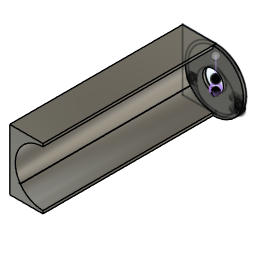
Sin+título(1) (Autodesk Fusion 360 design; units mm, degrees)
Autodesk Fusion 360 part; units mm, degrees
sketch "Boceto1" plane through (0, 0, 0) normal (0, 1, 0) x (1, 0, 0)
  circle A0 centre (0, 0) radius 14
  circle A1 centre (-17.5, 0) radius 2
  circle A2 centre (-17.5, 0) radius 3.5
  line L0 (-17.5, -3.5) -> (-13.5554, -3.5)
  line L1 (-17.5, 3.5) -> (-13.5554, 3.5)
  line L2 (0, -1.75) -> (0, -22.5)
  circle A3 centre (17.5, 0) radius 2
  circle A4 centre (17.5, 0) radius 3.5
  line L3 (17.5, 3.5) -> (13.5554, 3.5)
  line L4 (17.5, -3.5) -> (13.5554, -3.5)
  circle A5 centre (0, -8) radius 7.5
  circle A6 centre (0, -8) radius 20
  circle A7 centre (0, -8) radius 22
  line L5 (0, -30) -> (-24, -30)
  line L6 (-24, -30) -> (-24, 14)
  line L7 (-24, 14) -> (0, 14)
  line L8 (0, -30) -> (0, -28)
  line L9 (0, 14) -> (0, 12)
  dimension "d1" = 28
  dimension "d2" = 4
  dimension "d3" = 7
  dimension "d4" = 17.5
  dimension "d6" = 15
  dimension "d7" = 8
  dimension "d8" = 40
  dimension "d9" = 2
  dimension "d10" = 24
  constraint coincident A0.centre origin
  constraint concentric A1 A2
  constraint horizontal A0.centre A1.centre
  constraint coincident A2 L0.start
  constraint coincident A0 L0.end
  constraint coincident A2 L1.start
  constraint coincident A0 L1.end
  constraint tangent A2 L0
  constraint tangent A2 L1
  constraint horizontal L0
  constraint horizontal L1
  constraint symmetric A1 L2 A3
  constraint symmetric A2 L2 A4
  constraint symmetric L0.start L2 L4.start
  constraint symmetric L0.end L2 L4.end
  constraint symmetric L1.start L2 L3.start
  constraint symmetric L1.end L2 L3.end
  constraint vertical A0.centre A5.centre
  constraint concentric A5 A6
  constraint concentric A5 A7
  constraint coincident A7 L5.start
  constraint tangent A7 L5
  constraint perpendicular L5 L6
  constraint coincident A7 L7.end
  constraint tangent A7 L7
  constraint horizontal L7
  constraint horizontal L5
  constraint coincident A6 L8.end
  constraint perpendicular L5 L8
  constraint coincident A6 L9.end
  constraint perpendicular L7 L9
  measures "d1" diameter of A0
  measures "d2" diameter of A1
  measures "d3" diameter of A2
  measures "d4" distance of A0.centre A1.centre
  measures "d6" diameter of A5
  measures "d7" distance of A0.centre A5.centre
  measures "d8" diameter of A6
  measures "d9" distance of A6 A7
  measures "d10" horizontal distance of L5.start L5.end
extrude "Extruir1" add sketch "Boceto1" against normal blind 2 contours A0 A5 A6 | A0 A4 L4 | A3 A4 A6 | A0 A4 L3 A6 | A0 L3 A6 | A0 A2 L0 A4 L4 A5 A6 | A3 A4 A6 A7 | A0 A6 L9 | A0 A4 L3 A6 A7 | A4 A6 A7 L8 | A3 A6 | A3 A6 | A0 A6 L9 | A0 A2 L1 A6 A7 | A2 A7 L5 L6 L7 | A0 L1 A6 | A2 A7 | A1 A2 A6 A7 | A2 A6 A7 L8 | A0 A2 L1 A6 | A0 A2 L0 | A1 A2 A6 | A1 A6 | A1 A6
extrude "Extruir2" add sketch "Boceto1" against normal blind 125 contours A0 A6 L9 | A0 A2 L1 A6 A7 | A2 A7 L5 L6 L7 | A2 A7 | A1 A2 A6 A7 | A2 A6 A7 L8 | A1 A6 picked at (-1.6542, 12.5453) picked at (-18.5384, 0.5277)
equation "d4 = ( 35 / 2 ) * 1 mm"
